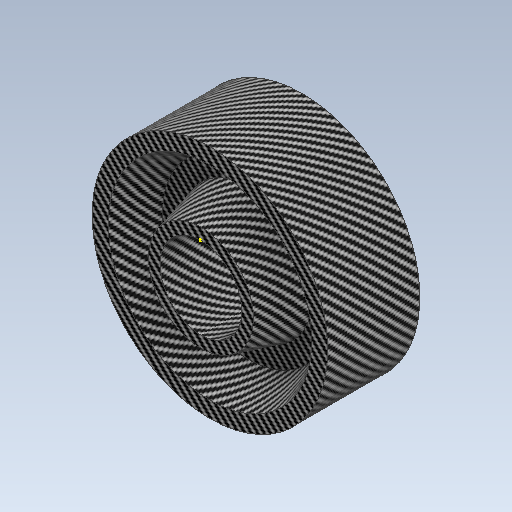
# Autodesk Inventor part: Part3
Saved by Autodesk Inventor 2021 (Build 250183000, 183)
## iProperties
Created: 2022-04-30
Part Number: Part3
Material: Iron, Cast
Document SubType Name: Modeling
Designer: authe
Density: 7.15 g/cm^3
Appearance: Carbon Fiber
Author: authe
Autodesk Inventor part; units mm, degrees
ref_plane "YZ Plane" through (0, 0, 0) normal (1, 0, 0) x (0, 1, 0)
ref_plane "XZ Plane" through (0, 0, 0) normal (0, 1, 0) x (-1, 0, 0)
ref_plane "XY Plane" through (0, 0, 0) normal (0, 0, 1) x (1, 0, 0)
sketch "Sketch1" plane through (0, 0, 0) normal (1, 0, 0) x (0, 1, 0)
  line L0 (0, 0) -> (0, -43)
  line L1 (0, -43) -> (4.5, -43)
  line L2 (0, 0) -> (4.5, 0)
  line L3 (4.5, 0) -> (0, 0)
  line L4 (0, 0) -> (30, 0)
  line L5 (30, 0) -> (25.5, 0)
  line L6 (25.5, 0) -> (30, 0)
  line L7 (30, 0) -> (30, -3.5)
  line L8 (30, -3.5) -> (30, -39.5)
  line L9 (30, -39.5) -> (30, -43)
  line L10 (23.7723, -3.5) -> (30, -3.5)
  line L11 (30, -39.5) -> (23.7723, -39.5)
  line L12 (23.7723, -39.5) -> (18.5312, -28.2604)
  line L13 (23.7723, -39.5) -> (36.1738, -39.5) construction
  line L14 (4.5, -43) -> (8.4495, -28.2604)
  line L15 (4.5, -43) -> (19.7596, -43) construction
  line L16 (0, 0) -> (0, -21.5)
  line L17 (0, -21.5) -> (30, -21.5)
  line L18 (18.5312, -28.2604) -> (17.0108, -25)
  line L19 (0, -21.5) -> (0, -21.5)
  line L20 (0, -21.5) -> (0, -25)
  line L21 (0, -25) -> (0, -18)
  line L22 (9.3236, -25) -> (17.0108, -25)
  line L23 (23.7723, -3.5) -> (17.0108, -18)
  line L24 (17.0108, -18) -> (9.3236, -18)
  line L25 (9.3236, -18) -> (4.5, 0)
  line L26 (9.3236, -25) -> (8.2254, -29.0967)
  line L27 (0, -43) -> (-16, -43)
  line L28 (-16, -43) -> (-16, -23.25)
  dimension "d0" = 43
  dimension "d1" = 4.5
  dimension "d2" = 4.5
  dimension "d3" = 30
  dimension "d4" = 4.5
  dimension "d5" = 3.5
  dimension "d6" = 36
  dimension "d7" = 3.5
  dimension "d8" = 115
  dimension "d9" = 75
  dimension "d11" = 21.5
  dimension "d12" = 0
  dimension "d13" = 3.5
  dimension "d14" = 7
  dimension "d29" = 25
  dimension "d30" = 25
  dimension "d31" = 15.006
  dimension "d32" = 15.001
  dimension "d33" = 14.5
  dimension "d34" = 3.5
  dimension "d35" = 4.8516
  dimension "d36" = 23.0242
  dimension "d37" = 15.4786
  dimension "d38" = 6.1738
  dimension "d39" = 10.2404
  dimension "d40" = 16
  constraints: 58 end point, 7 horizontal, 7 point on line, 3 midpoint, 2 collinear, 2 equal length, 2 perpendicular, 2 vertical, 1 parallel
  measures "d0" distance of L0.start L0.end
  measures "d1" distance of L0.end L1.end
  measures "d2" distance of L0.start L2.end
  measures "d3" distance of L0.start L4.end
  measures "d4" distance of L4.end L5.end
  measures "d5" distance of L4.end L7.end
  measures "d6" distance of L7.end L8.end
  measures "d7" distance of L8.end L9.end
  measures "d8" angle of L13 L12
  measures "d9" angle of L15 L14
  measures "d11" distance of L0.start L16.end
  measures "d12" distance of L16.end L19.end
  measures "d13" distance of L16.end L20.end
  measures "d14" distance of L20.end L21.end
  measures "d29" angle of L23 L8
  measures "d30" angle of L18 L8
  measures "d31" angle of L26 L8
  measures "d32" angle of L25 L8
  measures "d33" distance between parallel lines of L22 L13
  measures "d34" distance between parallel lines of L24 L17
  measures "d35" distance from line of L0.start L12
  measures "d36" distance from line of L0.start L23
  measures "d37" distance from line of L0.start L26
  measures "d38" distance from line of L13.end L8
  measures "d39" distance from line of L15.end L8
  measures "d40" distance of L0.end L27.end
sketch "Sketch2" plane through (0, 0, 0) normal (0, 1, 0) x (-1, 0, 0)
  point P0 (0, 0)
sketch "Sketch3" plane through (0, 0, 0) normal (1, 0, 0) x (0, 1, 0)
  line L0 (-16, -42.9893) -> (-16, -42.9893)
  line L1 (0, 0) -> (0, -42.9893)
  line L2 (0, -42.9893) -> (-16, -42.9893)
  dimension "d16" = 0
  constraints: 6 end point, 1 perpendicular, 1 vertical
  measures "d16" distance of L0.start L0.end
sketch "Sketch4" plane through (0, 0, 0) normal (1, 0, 0) x (0, 1, 0)
  line L0 (-16, 5.5421) -> (-16, 5.5421)
  line L1 (-16, -17.3048) -> (-16, -42.7531)
  point P0 (0, 0)
  dimension "d17" = 0
  constraints: 4 end point, 1 horizontal, 1 vertical
  measures "d17" distance of L0.start L0.end
revolve "Revolution1" add sketch "Sketch1" angle 360 about axis through (0, -16, -43) along (0, 0, 1) contours L2 L25 L24 L23 L10 L8 L17 L0 | L17 L8 L11 L12 L18 L22 L26 L14 L1 L0
body "Solid1"
